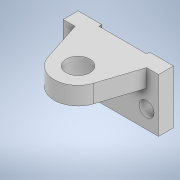
# Autodesk Inventor part: 零件2
Saved by Autodesk Inventor 2020 (Build 240168000, 168)
## iProperties
Created: 2023-11-09
Part Number: 零件2
Material: 常规
Document SubType Name: Modeling
Designer: Z
Density: 1 g/cm^3
Appearance: 默认
Author: Z
Autodesk Inventor part; units mm, degrees
ref_plane "YZ Plane" through (0, 0, 0) normal (1, 0, 0) x (0, 1, 0)
ref_plane "XZ Plane" through (0, 0, 0) normal (0, 1, 0) x (-1, 0, 0)
ref_plane "XY Plane" through (0, 0, 0) normal (0, 0, 1) x (1, 0, 0)
sketch "草图1" plane through (0, 0, 0) normal (0, 0, 1) x (1, 0, 0)
  line L0 (-16, 9) -> (16, 9)
  line L1 (16, 9) -> (16, -9)
  line L2 (16, -9) -> (-16, -9)
  line L3 (-16, -9) -> (-16, 9)
  line L4 (-16, 9) -> (16, -9) construction
  line L5 (16, 9) -> (-16, -9) construction
  circle A0 centre (-12, -3) radius 2.5
  circle A1 centre (12, -3) radius 2.5
  line L6 (-8, 9) -> (8, 9)
  line L7 (8, 9) -> (8, -9)
  line L8 (8, -9) -> (-8, -9)
  line L9 (-8, -9) -> (-8, 9)
  line L10 (-8, 9) -> (8, -9) construction
  line L11 (8, 9) -> (-8, -9) construction
  point P0 (0, 0)
  dimension "d0" = 32
  dimension "d1" = 18
  dimension "d2" = 5
  dimension "d3" = 12
  dimension "d4" = 4
  dimension "d5" = 5
  dimension "d6" = 12
  dimension "d7" = 4
  dimension "d8" = 16
  dimension "d9" = 18
  constraints: 24 end point, 4 midpoint, 4 parallel, 2 centre point, 2 horizontal, 2 perpendicular
  measures "d0" distance of L1.end L2.end
  measures "d1" distance of L0.end L1.end
  measures "d2" diameter of A0
  measures "d3" distance from line of L0 A0.centre
  measures "d4" distance from line of L3 A0.centre
  measures "d5" diameter of A1
  measures "d6" distance from line of L0 A1.centre
  measures "d7" distance from line of L1 A1.centre
  measures "d8" distance of L7.end L8.end
  measures "d9" distance of L6.end L7.end
extrude "拉伸1" add sketch "草图1" along normal blind 5
sketch "草图2" plane through (0, 0, 0) normal (0, 0, -1) x (-1, 0, 0)
  line L0 (8, -9) -> (-8, -9)
  line L1 (-8, -9) -> (-8, 9)
  line L2 (-8, 9) -> (8, 9)
  line L3 (8, 9) -> (8, -9)
  line L4 (8, -9) -> (-8, 9) construction
  line L5 (-8, -9) -> (8, 9) construction
  point P0 (0, 0)
  dimension "d12" = 16
  dimension "d13" = 18
  constraints: 12 end point, 2 midpoint, 2 parallel, 1 horizontal, 1 perpendicular
  measures "d12" distance of L1.end L2.end
  measures "d13" distance of L0.end L1.end
extrude "拉伸2" cut sketch "草图2" against normal blind 1
sketch "草图3" plane through (-16, 9, 5) normal (0, 1, 0) x (1, 0, 0)
  circle A0 centre (16, -11) radius 4
  arc A1 (8.3939, -13.4794) -> (23.6061, -13.4794) centre (16, -11) ccw
  line L0 (28, 0) -> (23.6061, -13.4794)
  line L1 (8.3939, -13.4794) -> (4, 0)
  line L2 (16, 5) -> (16, -11) construction
  line L3 (32, 0) -> (0, 0) projected
  line L4 (28, 0) -> (4, 0)
  dimension "d16" = 8
  dimension "d18" = 8
  dimension "d19" = 24
  dimension "d21" = 16
  dimension "d22" = 18.055
  dimension "d23" = 36.109
  dimension "d24" = 12
  constraints: 8 end point, 2 centre point, 2 point on circle, 2 tangent, 1 coincident, 1 vertical
  measures "d16" diameter of A0
  measures "d18" radius of A1
  measures "d19" distance of L1.end L0.start
  measures "d21" distance of L2.start A0.centre
  measures "d22" angle of L0 L2
  measures "d23" angle of L0 L1
  measures "d24" distance from line of L0.start L2
extrude "拉伸3" add sketch "草图3" against normal blind 6
